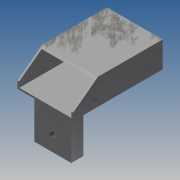
# Autodesk Inventor part: 2p0hh
Saved by Autodesk Inventor 2013 (Build 170138000, 138)
## iProperties
Company: HERA Project
Created: 2013-12-03
Part Number: 2p0hh
Material: Steel, Galvanized
Document SubType Name: Modeling
Designer: David DeBoer
Mass: 1619.54 g
Surface Area: 865.184 cm^2
Volume: 206.311 cm^3
Density: 7.85 g/cm^3
Description: end horizontal holder
Author: David DeBoer
Autodesk Inventor part; units mm, degrees
ref_plane "YZ Plane" through (0, 0, 0) normal (1, 0, 0) x (0, 1, 0)
ref_plane "XZ Plane" through (0, 0, 0) normal (0, 1, 0) x (-1, 0, 0)
ref_plane "XY Plane" through (0, 0, 0) normal (0, 0, 1) x (1, 0, 0)
sketch "Sketch1" plane through (0, 0, 0) normal (0, 0, 1) x (1, 0, 0)
  line L0 (0, 0) -> (88.9, 0)
  line L1 (88.9, 0) -> (88.9, 38.1)
  line L2 (88.9, 38.1) -> (0, 38.1)
  line L3 (0, 38.1) -> (0, 0)
  line L4 (-3.048, 41.148) -> (91.948, 41.148)
  line L5 (91.948, 41.148) -> (91.948, -3.048)
  line L6 (91.948, -3.048) -> (-3.048, -3.048)
  line L7 (-3.048, -3.048) -> (-3.048, 41.148)
  dimension "d0" = 88.9
  dimension "d1" = 38.1
  dimension "d2" = 3.048
  constraints: 16 end point, 4 parallel, 2 perpendicular, 1 horizontal, 3 other
  measures "d0" distance of L0.start L0.end
  measures "d1" distance of L2.end L0.start
  measures "d2" distance between parallel lines of L4 L2
extrude "Extrusion1" add sketch "Sketch1" along normal blind 152.4
ref_plane "Work Plane1" through (-3.048, 41.148, 152.4) normal (0, 0.7986355, 0.601815) x (-1, 0, 0)
sketch "Sketch2" plane through (-3.048, 41.148, 152.4) normal (0, 0.7986355, 0.601815) x (-1, 0, 0)
  line L0 (-144.4625, 77.7875) -> (65.0875, 77.7875)
  line L1 (65.0875, 77.7875) -> (65.0875, -49.2125)
  line L2 (65.0875, -49.2125) -> (-144.4625, -49.2125)
  line L3 (-144.4625, -49.2125) -> (-144.4625, 77.7875)
  point P0 (-3.048, -96.9486)
  dimension "d8" = 127
  constraints: 8 end point, 2 parallel, 1 horizontal, 1 perpendicular
  measures "d8" distance of L2.end L0.start
extrude "Extrusion2" cut sketch "Sketch2" against normal blind 25.4
sketch "Sketch3" plane through (-3.048, -3.048, 0) normal (0, -1, 0) x (1, 0, 0)
  line L0 (94.996, 0) -> (0, 0) projected
  line L1 (0, 152.4) -> (94.996, 152.4) projected
  line L2 (15.875, 119.0625) -> (79.121, 119.0625)
  line L3 (79.121, 119.0625) -> (79.121, 139.7)
  line L4 (79.121, 139.7) -> (15.875, 139.7)
  line L5 (15.875, 139.7) -> (15.875, 119.0625)
  line L6 (47.498, 139.7) -> (47.498, 119.0625) construction
  line L7 (47.498, 152.4) -> (47.498, 0) construction
  line L8 (15.875, 129.3812) -> (79.121, 129.3813) construction
  point P0 (3.048, 0)
  dimension "d10" = 12.7
  constraints: 14 end point, 6 midpoint, 2 parallel, 1 collinear, 1 horizontal, 1 perpendicular
  measures "d10" distance between parallel lines of L4 L1
extrude "Extrusion3" add sketch "Sketch3" along normal blind 76.2
sketch "Sketch4" plane through (12.827, -3.048, 139.7) normal (0, 0, 1) x (1, 0, 0)
  line L0 (63.246, -76.2) -> (0, -76.2) projected
  circle A0 centre (31.623, -50.8) radius 3.6638
  point P0 (-12.827, 3.048)
  dimension "d13" = 25.4
  constraints: 1 centre point
  measures "d13" distance from line of A0.centre L0
hole "Hole1" at (44.45, -53.848, 139.7) direction (0, 0, -1) diameter 10.5918 end through all thread size "1/2-13 UNC" class "2B" standard "ANSI Unified Screw Threads"
body "Solid1"
